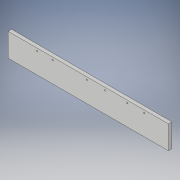
# Autodesk Inventor part: Kermit bumper (middle 4)
Saved by Autodesk Inventor 2018.2 (Build 222227000, 227)
## iProperties
Created: 2018-02-15
Part Number: Kermit bumper (middle 4)
Material: Generic
Document SubType Name: Modeling
Designer: kalra.rohan
Density: 1 g/cm^3
Appearance: Default
Author: kalra.rohan
Autodesk Inventor part; units mm, degrees
ref_plane "YZ Plane" through (0, 0, 0) normal (1, 0, 0) x (0, 1, 0)
ref_plane "XZ Plane" through (0, 0, 0) normal (0, 1, 0) x (-1, 0, 0)
ref_plane "XY Plane" through (0, 0, 0) normal (0, 0, 1) x (1, 0, 0)
sketch "Sketch1" plane through (0, 0, 0) normal (0, 0, 1) x (1, 0, 0)
  line L0 (0, 0) -> (831.85, 0)
  line L1 (831.85, 0) -> (831.85, -120.65)
  line L2 (831.85, -120.65) -> (0, -120.65)
  line L3 (0, -120.65) -> (0, 0)
  circle A0 centre (150.5966, -13.462) radius 3.556
  circle A1 centre (230.8606, -13.462) radius 3.556
  circle A2 centre (408.6606, -13.462) radius 3.556
  circle A3 centre (503.5296, -13.462) radius 3.556
  circle A4 centre (618.0836, -13.462) radius 3.556
  circle A5 centre (706.7296, -13.462) radius 3.556
  dimension "d0" = 831.85
  dimension "d1" = 120.65
  dimension "d2" = 7.112
  dimension "d3" = 150.5966
  dimension "d4" = 107.188
  dimension "d5" = 7.112
  dimension "d6" = 80.264
  dimension "d7" = 107.188
  dimension "d8" = 7.112
  dimension "d9" = 107.188
  dimension "d10" = 177.8
  dimension "d11" = 7.112
  dimension "d12" = 107.188
  dimension "d13" = 94.869
  dimension "d14" = 7.112
  dimension "d15" = 107.188
  dimension "d16" = 114.554
  dimension "d17" = 7.112
  dimension "d19" = 88.646
  dimension "d20" = 107.188
  constraints: 8 end point, 6 centre point, 2 parallel, 1 horizontal, 1 perpendicular
  measures "d0" distance between parallel lines of L1 L3
  measures "d1" distance between parallel lines of L2 L0
  measures "d2" diameter of A0
  measures "d3" distance from line of A0.centre L3
  measures "d4" distance from line of A0.centre L2
  measures "d5" diameter of A1
  measures "d6" distance of A1.centre A0.centre
  measures "d7" distance from line of A1.centre L2
  measures "d8" diameter of A2
  measures "d9" distance from line of A2.centre L2
  measures "d10" distance of A2.centre A1.centre
  measures "d11" diameter of A3
  measures "d12" distance from line of A3.centre L2
  measures "d13" distance of A3.centre A2.centre
  measures "d14" diameter of A4
  measures "d15" distance from line of A4.centre L2
  measures "d16" distance of A4.centre A3.centre
  measures "d17" diameter of A5
  measures "d19" distance of A5.centre A4.centre
  measures "d20" distance from line of A5.centre L2
extrude "Extrusion1" add sketch "Sketch1" against normal blind 18.3261
body "Solid1"
